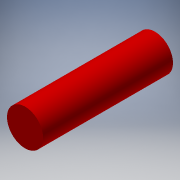
# Autodesk Inventor part: Short Noodle
Saved by Autodesk Inventor 2018 (Build 220112000, 112)
## iProperties
Created: 2018-01-17
Part Number: Short Noodle
Material: Generic
Document SubType Name: Modeling
Designer: Apple
Density: 1 g/cm^3
Appearance: Default
Author: Apple
Autodesk Inventor part; units mm, degrees
ref_plane "YZ Plane" through (0, 0, 0) normal (1, 0, 0) x (0, 1, 0)
ref_plane "XZ Plane" through (0, 0, 0) normal (0, 1, 0) x (-1, 0, 0)
sketch "Sketch1" plane through (0, 0, 0) normal (0, 0, 1) x (1, 0, 0)
  circle A0 centre (96.0333, 50.0167) radius 30.9667
  line L0 (0, 19.05) -> (127, 19.05) projected
  line L1 (127, 0) -> (127, 19.05) projected
  line L2 (127, 0) -> (127, 102.2315) construction
  point P0 (0, 0)
  constraints: 2 end point, 2 tangent, 1 centre point, 1 vertical
ref_plane "Work Plane1" through (0, 0, -158.75) normal (0, 0, -1) x (0, 1, 0)
extrude "Extrusion1" add sketch "Sketch1" against normal blind 158.75 and the other way blind 63.5
body "Solid1"
